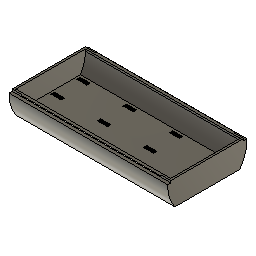
bottom log final prototype (Autodesk Fusion 360 design; units mm, degrees)
part number: 2026-03-30-13-21-05-084
Autodesk Fusion 360 part; units mm, degrees
note: some values were not read from the file. Set by a fixed rule: which sketch regions a step uses.
sketch "Sketch2" plane through (0, 0, 0) normal (1, 0, 0) x (0, 1, 0)
  line L0 (-50.8, 0) -> (-44.45, 0)
  line L1 (44.45, 0) -> (50.8, 0)
  line L2 (-44.45, 0) -> (-44.45, 2.54)
  line L3 (-44.45, 2.54) -> (-48.006, 2.54)
  line L4 (-48.006, 2.54) -> (-46.736, 0)
  line L5 (0, 2.5) -> (0, 20)
  line L6 (48.006, 2.54) -> (46.736, 0)
  line L7 (44.45, 2.54) -> (48.006, 2.54)
  line L8 (44.45, 0) -> (44.45, 2.54)
  line L9 (38.1212, -22.86) -> (-38.1212, -22.86)
  line L10 (41.5622, -29.21) -> (-41.5622, -29.21)
  arc A0 (-50.8, 0) -> (-41.5622, -29.21) centre (0, 0) ccw
  arc A1 (41.5622, -29.21) -> (50.8, 0) centre (0, 0) ccw
  arc A2 (-44.45, 0) -> (-38.1212, -22.86) centre (0, 0) ccw
  arc A3 (38.1212, -22.86) -> (44.45, 0) centre (0, 0) ccw
  dimension "d5" = 101.6
  dimension "d6" = 88.9
  dimension "d7" = 101.6
  dimension "d8" = 4.064
  dimension "d9" = 2.54
  dimension "d10" = 3.556
  dimension "d18" = 25.4
  dimension "d19" = 6.35
  dimension "d20" = 44.45
  constraint coincident A0.centre A1.centre
  constraint horizontal L0
  constraint collinear L0 L1
  constraint tangent L2 A2
  constraint perpendicular L2 L3
  constraint coincident L0 L4.end
  constraint symmetric L0.end L5 L1.start
  constraint symmetric L2.end L5 L7.start
  constraint symmetric L3.end L5 L6.start
  constraint symmetric L4.end L5 L6.end
  constraint horizontal L9
  constraint horizontal L10
  constraint concentric A0 A1
  constraint concentric A2 A3
  measures "d5" diameter of A0
  measures "d6" diameter of A2
  measures "d7" distance of L0.start L1.end
  measures "d8" distance of L0.start L4.end
  measures "d9" distance of L0.end L2.end
  measures "d10" distance of L2.end L3.end
  measures "d18" distance of L3 L9
  measures "d19" distance of L9 L10
  measures "d20" radius of A3
extrude "Extrude1" add sketch "Sketch2" along normal mid plane 203.2
sketch "Sketch4" plane through (101.6, 0, 0) normal (1, 0, 0) x (0, 1, 0)
  line L0 (46.736, 0) -> (48.006, 2.54)
  line L1 (48.006, 2.54) -> (44.45, 2.54)
  line L2 (44.45, 2.54) -> (44.45, 0)
  arc A0 (38.1212, -22.86) -> (44.45, 0) centre (0, 0) ccw
  line L3 (38.1212, -22.86) -> (-38.1212, -22.86)
  arc A1 (-44.45, 0) -> (-38.1212, -22.86) centre (0, 0) ccw
  line L4 (-44.45, 0) -> (-44.45, 2.54)
  line L5 (-44.45, 2.54) -> (-48.006, 2.54)
  line L6 (-48.006, 2.54) -> (-46.736, 0)
  line L7 (-46.736, 0) -> (-50.8, 0)
  arc A2 (-50.8, 0) -> (-41.5622, -29.21) centre (0, 0) ccw
  line L8 (-41.5622, -29.21) -> (41.5622, -29.21)
  arc A3 (41.5622, -29.21) -> (50.8, 0) centre (0, 0) ccw
  line L9 (50.8, 0) -> (46.736, 0)
  line L10 (-44.45, 2.54) -> (44.45, 2.54)
  constraint coincident L4.end L5.start
  constraint coincident L1.end L2.start
extrude "Extrude3" add sketch "Sketch4" against normal blind 2.54
mirror "Mirror2" about plane through (0, 0, 0) normal (1, 0, 0) of "Extrude3"
sketch "Sketch5" plane through (101.6, 0, 0) normal (1, 0, 0) x (0, 1, 0)
  line L0 (46.736, 0) -> (48.006, 2.54)
  line L1 (48.006, 2.54) -> (-48.006, 2.54)
  line L2 (-48.006, 2.54) -> (-46.736, 0)
  line L3 (-46.736, 0) -> (-50.8, 0)
  arc A0 (-50.8, 0) -> (-41.5622, -29.21) centre (0, 0) ccw
  line L4 (-41.5622, -29.21) -> (41.5622, -29.21)
  arc A1 (41.5622, -29.21) -> (50.8, 0) centre (0, 0) ccw
  line L5 (50.8, 0) -> (46.736, 0)
  line L6 (-46.736, 0) -> (-49.276, 0)
  line L7 (-49.276, 0) -> (-49.276, 2.54)
  line L8 (-49.276, 2.54) -> (-46.736, 2.54)
  line L9 (-46.736, 2.54) -> (-46.736, 0)
  dimension "d25" = 2.54
  dimension "d26" = 2.54
  constraint horizontal L6
  constraint vertical L7
  constraint horizontal L8
  constraint vertical L9
  constraint coincident L2.end L3.start
  measures "d25" distance of L6.end L7.end
  measures "d26" distance of L7.end L8.end
extrude "Extrude4" cut sketch "Sketch5" against normal blind 12.7 contours L1 L2 L8 L9 | L2 L3 L6 L7 L8
mirror "Mirror3" about plane through (0, 0, 0) normal (0, 1, 0) of "Extrude4"
mirror "Mirror4" about plane through (0, 0, 0) normal (1, 0, 0) of "Extrude4"
sketch "Sketch6" plane through (0, 0, -29.21) normal (0, 0, -1) x (1, 0, 0)
  line L0 (-101.6, -41.5622) -> (101.6, -41.5622)
  line L1 (101.6, -41.5622) -> (101.6, 41.5622)
  line L2 (101.6, 41.5622) -> (-101.6, 41.5622)
  line L3 (-101.6, 41.5622) -> (-101.6, -41.5622)
  line L4 (-96.52, 35.2122) -> (-83.82, 35.2122)
  line L5 (-83.82, 35.2122) -> (-83.82, 34.7042)
  line L6 (-83.82, 34.7042) -> (-96.52, 34.7042)
  line L7 (-96.52, 34.7042) -> (-96.52, 35.2122)
  dimension "d33" = 0.508
  dimension "d34" = 12.7
  dimension "d35" = 6.35
  constraint horizontal L4
  constraint vertical L5
  constraint horizontal L6
  constraint vertical L7
  measures "d33" distance of L4.end L5.end
  measures "d34" distance of L4.start L4.end
  measures "d35" distance of L2 L4
extrude "Extrude5" cut sketch "Sketch6" against normal through all contours L4 L5 L6 L7
pattern_linear "R-Pattern1" count 5 spacing 0.9525 along (0, 1, 0) of "Extrude5"
pattern_linear "R-Pattern2" count 3 spacing 33.02 along (0, 1, 0) of "Extrude5", "R-Pattern1"
pattern_linear "R-Pattern3" count 4 spacing 59.2667 along (1, 0, 0) of "Extrude5", "R-Pattern1", "R-Pattern2"
mirror "Mirror5" about plane through (0, 0, 0) normal (0, 1, 0) of "Mirror4"
